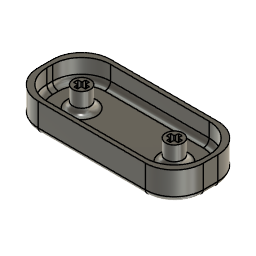
EnterKeycap (Autodesk Fusion 360 design; units mm, degrees)
Autodesk Fusion 360 part; units mm, degrees
sketch "Sketch1" plane through (0, 0, 0) normal (0, 0, 1) x (1, 0, 0)
  line L0 (-28.5, 12.5) -> (28.5, 12.5)
  line L1 (28.5, 12.5) -> (28.5, -12.5)
  line L2 (28.5, -12.5) -> (-28.5, -12.5)
  line L3 (-28.5, -12.5) -> (-28.5, 12.5)
  dimension "d1" = 25
  dimension "d2" = 57
  dimension "d3" = 12.5
  dimension "d4" = 28.5
  constraint horizontal L0
  constraint vertical L1
  constraint horizontal L2
  constraint vertical L3
  measures "d1" distance of L0.start L2.end
  measures "d2" distance of L0.start L0.end
  measures "d3" vertical distance of origin L0.start
  measures "d4" horizontal distance of origin L0.end
extrude "Extrude1" add sketch "Sketch1" along normal blind 3 makes body 1
sketch "Sketch2" plane through (0, 0, 3) normal (0, 0, 1) x (-1, 0, 0)
  line L0 (28.5, 12.5) -> (-28.5, 12.5)
  line L1 (-28.5, 12.5) -> (-28.5, -12.5)
  line L2 (-28.5, -12.5) -> (28.5, -12.5)
  line L3 (28.5, -12.5) -> (28.5, 12.5)
  line L4 (28.5, -12.5) -> (-28.5, -12.5)
  line L5 (-28.5, -12.5) -> (-28.5, 12.5)
  line L6 (-28.5, 12.5) -> (28.5, 12.5)
  line L7 (28.5, 12.5) -> (28.5, -12.5)
  line L8 (27, -11) -> (-27, -11)
  line L9 (-27, -11) -> (-27, 11)
  line L10 (-27, 11) -> (27, 11)
  line L11 (27, 11) -> (27, -11)
  line L12 (16.6, -2) -> (15.4, -2)
  line L13 (16.6, -1) -> (16.6, -2)
  arc A0 (-16.9, 0.7) -> (-16.6, 1) centre (-16.9, 1) ccw
  line L14 (14, -0.7) -> (14, 0.7)
  line L15 (-18, 0.7) -> (-16.9, 0.7)
  line L16 (-16.6, 1) -> (-16.6, 2)
  line L17 (-18, -0.7) -> (-18, 0.7)
  arc A1 (15.4, -1) -> (15.1, -0.7) centre (15.1, -1) ccw
  circle A2 centre (-16, 0) radius 3
  line L18 (-15.4, 2) -> (-15.4, 1)
  line L19 (14, 0.7) -> (15.1, 0.7)
  line L20 (-14, 0.7) -> (-14, -0.7)
  arc A3 (-16.6, -1) -> (-16.9, -0.7) centre (-16.9, -1) ccw
  line L21 (15.4, 2) -> (16.6, 2)
  line L22 (-15.4, -2) -> (-16.6, -2)
  line L23 (-16.9, -0.7) -> (-18, -0.7)
  line L24 (18, -0.7) -> (16.9, -0.7)
  arc A4 (-15.1, -0.7) -> (-15.4, -1) centre (-15.1, -1) ccw
  circle A5 centre (16, 0) radius 3
  line L25 (15.1, -0.7) -> (14, -0.7)
  arc A6 (16.9, -0.7) -> (16.6, -1) centre (16.9, -1) ccw
  line L26 (-16.6, 2) -> (-15.4, 2)
  line L27 (-15.1, 0.7) -> (-14, 0.7)
  line L28 (-15.4, -1) -> (-15.4, -2)
  line L29 (16.6, 2) -> (16.6, 1)
  line L30 (-14, -0.7) -> (-15.1, -0.7)
  arc A7 (-15.4, 1) -> (-15.1, 0.7) centre (-15.1, 1) ccw
  line L31 (15.4, 1) -> (15.4, 2)
  line L32 (15.4, -2) -> (15.4, -1)
  arc A8 (16.6, 1) -> (16.9, 0.7) centre (16.9, 1) ccw
  arc A9 (15.1, 0.7) -> (15.4, 1) centre (15.1, 1) ccw
  line L33 (-16.6, -2) -> (-16.6, -1)
  line L34 (18, 0.7) -> (18, -0.7)
  line L35 (16.9, 0.7) -> (18, 0.7)
  point P0 (-16, 0)
  point P1 (16, 0)
  point P2 (-15.4, 0.7)
  point P3 (16.6, 0.7)
  dimension "d7" = 1.5
  dimension "d8" = 1.5
  dimension "d9" = 1.5
  dimension "d10" = 1.5
  dimension "d11" = 4
  dimension "d12" = 4
  dimension "d13" = 2
  dimension "d14" = 2
  dimension "d15" = 1.2
  dimension "d16" = 1.4
  dimension "d17" = 0.7
  dimension "d18" = 0.6
  dimension "d19" = 0.3
  dimension "d20" = 6
  dimension "d21" = 4
  dimension "d22" = 4
  dimension "d23" = 2
  dimension "d24" = 2
  dimension "d25" = 1.2
  dimension "d26" = 1.4
  dimension "d27" = 0.7
  dimension "d28" = 0.6
  dimension "d29" = 0.3
  dimension "d30" = 6
  dimension "d31" = 32
  dimension "d32" = 16
  constraint horizontal L4
  constraint vertical L5
  constraint horizontal L6
  constraint vertical L7
  constraint coincident L0.end L1.start
  constraint coincident L2.end L3.start
  constraint horizontal L8
  constraint vertical L9
  constraint horizontal L10
  constraint vertical L11
  constraint vertical L16
  constraint perpendicular L16 L26
  constraint perpendicular L18 L26
  constraint perpendicular L18 L27
  constraint perpendicular L20 L27
  constraint perpendicular L20 L30
  constraint perpendicular L27 L28
  constraint perpendicular L22 L28
  constraint perpendicular L22 L33
  constraint perpendicular L23 L33
  constraint perpendicular L17 L22
  constraint perpendicular L15 L16
  constraint tangent A0 L16
  constraint tangent A0 L15
  constraint coincident P2 L18
  constraint coincident P2 L27
  constraint tangent L18 A7
  constraint tangent L27 A7
  constraint equal A0 A7
  constraint tangent A3 L33
  constraint tangent A3 L23
  constraint equal A0 A3
  constraint tangent A4 L30
  constraint tangent A4 L28
  constraint equal A0 A4
  constraint horizontal A0.start P2
  constraint horizontal A3.end A4.start
  constraint vertical A3.start A0.end
  constraint vertical A4.end P2
  constraint coincident P0 A2.centre
  constraint vertical L31
  constraint perpendicular L21 L31
  constraint perpendicular L21 L29
  constraint perpendicular L29 L35
  constraint perpendicular L34 L35
  constraint perpendicular L24 L34
  constraint perpendicular L13 L35
  constraint perpendicular L12 L13
  constraint perpendicular L12 L32
  constraint perpendicular L25 L32
  constraint perpendicular L12 L14
  constraint perpendicular L19 L31
  constraint tangent L31 A9
  constraint tangent L19 A9
  constraint coincident P3 L29
  constraint coincident P3 L35
  constraint tangent L29 A8
  constraint tangent A8 L35
  constraint equal A8 A9
  constraint tangent A1 L32
  constraint tangent A1 L25
  constraint equal A1 A9
  constraint tangent L24 A6
  constraint tangent L13 A6
  constraint equal A6 A9
  constraint horizontal L19.end P3
  constraint horizontal A1.end L24.end
  constraint vertical L31.start A1.start
  constraint vertical L13.start P3
  constraint coincident P1 A5.centre
  constraint horizontal P0 P1
  constraint horizontal origin P1
  measures "d7" distance of L4 L8
  measures "d8" distance of L6 L10
  measures "d9" distance of L7 L11
  measures "d10" distance of L5 L9
  measures "d11" distance of L17 L20
  measures "d12" distance of L22 L26
  measures "d13" distance of P0 L20
  measures "d14" distance of P0 L22
  measures "d15" distance of L18.start L16.end
  measures "d16" distance of L20.start L20.end
  measures "d17" vertical distance of P0 P2
  measures "d18" horizontal distance of P0 P2
  measures "d19" radius of A0
  measures "d20" diameter of A2
  measures "d21" distance of L14 L34
  measures "d22" distance of L12 L21
  measures "d23" distance of P1 L34
  measures "d24" distance of P1 L12
  measures "d25" distance of L21.start L21.end
  measures "d26" distance of L34.start L24.start
  measures "d27" vertical distance of P1 P3
  measures "d28" horizontal distance of P1 P3
  measures "d29" radius of A9
  measures "d30" diameter of A5
  measures "d31" distance of P0 P1
  measures "d32" distance of origin P1
extrude "Extrude2" add sketch "Sketch2" along normal blind 7 bodies 1
extrude "Extrude5" add 2 faces at (15.7655, 0.2578, 3) (-16.2345, -0.2578, 3) along direction (0, 0, 1) blind 3.3 on bodies 1 bodies 1
fillet "Fillet1" radius 10 8 edges at (28.5, 12.5, 5) (27, 11, 6.5) (27, -11, 6.5) (28.5, -12.5, 5) (-27, -11, 6.5) (-28.5, -12.5, 5) (-27, 11, 6.5) (-28.5, 12.5, 5) on bodies 1
fillet "Fillet1" radius 2 2 faces at (-4.968, -8.2642, 3) (-9.5, 4.1667, 0) on bodies 1
sketch "Sketch3" plane through (0, 0, 0) normal (0, 0, -1) x (1, 0, 0)
  arc A0 (18.5, -10.5) -> (26.5, -2.5) centre (18.5, -2.5) ccw
  line L0 (26.5, -2.5) -> (26.5, 2.5)
  arc A1 (26.5, 2.5) -> (18.5, 10.5) centre (18.5, 2.5) ccw
  line L1 (18.5, 10.5) -> (-18.5, 10.5)
  arc A2 (-18.5, 10.5) -> (-26.5, 2.5) centre (-18.5, 2.5) ccw
  line L2 (-26.5, 2.5) -> (-26.5, -2.5)
  arc A3 (-26.5, -2.5) -> (-18.5, -10.5) centre (-18.5, -2.5) ccw
  line L3 (-18.5, -10.5) -> (18.5, -10.5)
  line L4 (-3, -5) -> (-3, -1)
  line L5 (-3, -1) -> (5, -1)
  line L6 (5, -1) -> (5, -2.5)
  line L7 (5, -2.5) -> (9, 0)
  line L8 (9, 0) -> (5, 2.5)
  line L9 (5, 2.5) -> (5, 1)
  line L10 (5, 1) -> (-5, 1)
  line L11 (-5, 1) -> (-5, -5)
  line L12 (-5, -5) -> (-3, -5)
  dimension "d39" = 2
  dimension "d40" = 2
  dimension "d41" = 1.5
  dimension "d42" = 1.5
  dimension "d43" = 1
  dimension "d44" = 10
  dimension "d45" = 6
  dimension "d46" = 4
  dimension "d47" = 9
  dimension "d48" = 1
  constraint vertical L9
  constraint perpendicular L10 L11
  constraint horizontal L12
  constraint vertical L11
  constraint vertical L4
  constraint horizontal L5
  constraint vertical L6
  constraint vertical L5.end L9.end
  measures "d39" distance of L5 L10
  measures "d40" distance of L4 L11
  measures "d41" distance of L5.end L6.end
  measures "d42" distance of L8.end L9.end
  measures "d43" vertical distance of L5.end L7.end
  measures "d44" distance of L9.end L10.end
  measures "d45" distance of L10.end L12
  measures "d46" horizontal distance of L5.end L7.end
  measures "d47" horizontal distance of origin L7.end
  measures "d48" vertical distance of origin L10.end
extrude "Extrude3" cut sketch "Sketch3" against normal blind 0.4 contours L4 L5 L6 L7 L8 L9 L10 L11 L12 bodies 1
extrude "Extrude4" add 1 faces at (-1, -0.3333, 0.4) along direction (0, 0, -1) blind 0.4 separate body on bodies 1 makes body 2
equation "d3 = ( 25 / 2 ) * 1 mm"
equation "d4 = ( 57 / 2 ) * 1 mm"
